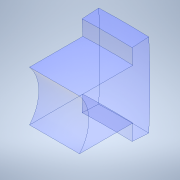
# Autodesk Inventor part: shank_2
Saved by Autodesk Inventor 2020.2 (Build 242310000, 310)
## iProperties
Created: 2021-01-30
Part Number: shank_2
Material: Generic
Document SubType Name: Modeling
Designer: DELL
Density: 1 g/cm^3
Appearance: Clear - Blue
Author: DELL
Autodesk Inventor part; units mm, degrees
ref_plane "XZ Plane" through (0, 0, 0) normal (0, 1, 0) x (-1, 0, 0)
ref_plane "XY Plane" through (0, 0, 0) normal (0, 0, 1) x (1, 0, 0)
ref_plane "UCS1: YZ Plane" through (0, 0, 0) normal (1, 0, 0) x (0, 1, 0)
sketch "Sketch17" plane through (0, 0, 0) normal (1, 0, 0) x (0, 1, 0)
  line L0 (-199.6617, 0) -> (149.874, 0) construction
  line L1 (0, -332.0076) -> (0, 872.0459) projected
  circle A0 centre (0, 0) radius 40
  circle A1 centre (0, 0) radius 46
  arc A2 (-58.5378, -97.8172) -> (58.5378, -97.8172) centre (0, 700.0382) ccw
  arc A3 (-60, -117.7468) -> (60, -117.7468) centre (0, 680) ccw
  line L2 (58.5378, -97.8172) -> (60, -117.7468)
  line L3 (-60, -117.7468) -> (-58.5378, -97.8172)
  line L4 (-30, -34.8712) -> (-30, -99.9618)
  line L5 (-30, -99.9618) -> (30, -99.9618)
  line L6 (30, -99.9618) -> (30, -34.8712)
  line L7 (-48.7654, -98.4741) -> (-50, -118.436)
  line L8 (48.7654, -98.4741) -> (50, -118.436)
  line L9 (-50, -118.436) -> (29.9324, -123.4415) construction
  line L10 (-48.7654, -98.4741) -> (31.1746, -103.3561) construction
  line L11 (-49.3827, -108.455) -> (42.5615, -114.1415) construction
  arc A4 (27.1283, -83.9618) -> (26, -99.9618) centre (99.9403, -97.1362) ccw
  arc A5 (27.1283, -83.9618) -> (30, -51.9618) centre (-149.7281, -51.9618) ccw
  point P0 (0, -120)
  point P1 (0, -99.9618)
  point P2 (0, -120)
  point P3 (0, -46)
  point P4 (0, -99.9618)
  dimension "d173" = 92
  dimension "d174" = 80
  dimension "d224" = 60
  dimension "d229" = 120
  dimension "d230" = 800
  dimension "d231" = 19.9831
  dimension "d232" = 100
  dimension "d233" = 10
  dimension "d235" = 800
  dimension "d241" = 20
  dimension "d242" = 18.7654
  dimension "d243" = 16
  dimension "d244" = 32
  dimension "d245" = 26
  constraints: 20 end point, 16 point on circle, 6 centre point, 5 tangent, 4 point on line, 3 perpendicular, 2 coincident, 1 equal length, 1 line through centre, 1 midpoint, 1 vertical, 5 other
  measures "d173" diameter of A1
  measures "d174" diameter of A0
  measures "d224" distance of L4.end L5.end
  measures "d229" distance from line of point (0, -120) L0
  measures "d230" radius of A3
  measures "d231" distance of L2.start L2.end
  measures "d232" diameter of L7.end L1
  measures "d233" horizontal distance of L3.start L7.end
  measures "d235" radius of A2
  measures "d241" distance of L8.start L8.end
  measures "d242" distance from line of L6 L8.start
  measures "d243" vertical distance of A4.end A4.start
  measures "d244" vertical distance of A4.start A5.end
  measures "d245" distance from line of A4.end L1
sketch "Sketch16" plane through (0, 0, 0) normal (1, 0, 0) x (0, 1, 0)
  circle A0 centre (0, 0) radius 40
  circle A1 centre (0, 0) radius 48.5
  line L0 (0, -201.7) -> (0, 90.2) construction
  line L1 (0, -160) -> (0, -48.5)
  line L2 (30, -38.1084) -> (30, -103.6436)
  line L3 (30, -103.6436) -> (25, -132)
  line L4 (25, -132) -> (50, -132)
  line L5 (50, -132) -> (50, -160)
  line L6 (50, -160) -> (0, -160)
  dimension "d156" = 97
  dimension "d157" = 80
  dimension "d202" = 28
  dimension "d203" = 60
  dimension "d204" = 50
  dimension "d206" = 160
  dimension "d209" = 50
  dimension "d210" = 80
  dimension "d211" = 28.7938
  constraints: 12 end point, 2 centre point, 2 coincident, 2 horizontal, 2 point on circle, 2 point on line, 2 vertical
  measures "d156" diameter of A1
  measures "d157" diameter of A0
  measures "d202" distance of L4.end L5.end
  measures "d203" diameter of L2 L0
  measures "d204" distance of L5.end L1.start
  measures "d206" distance from line of point (0, 0) L6
  measures "d209" diameter of L3.end L0
  measures "d210" angle of L4 L3
  measures "d211" distance of L2.end L3.end
revolve "Revolution2" add sketch "Sketch17" angle 360 about axis through (0, 0, -10) along (0, 0, 1) contours L1 L5 L6 A2 L8 A3 | A2 A4 L5 | L8 A2 L2 A3 | A2 L6 L5 A4
ref_plane "Work Plane7" through (0, -48.7654, -98.4741) normal (0, -0.998093, 0.0617284) x (0, -0.0617284, -0.998093)
split "Split2" plane through (0, -48.7654, -98.4741) removes the side toward (0, -0.998093, 0.0617284)
ref_plane "Work Plane8" through (0, 48.7654, -98.4741) normal (0, -0.998093, -0.0617284) x (0, 0.0617284, -0.998093)
split "Split3" plane through (0, 48.7654, -98.4741) removes the side toward (0, 0.998093, 0.0617284)
ref_plane "Work Plane9" through (-30, 0, 0) normal (1, 0, 0) x (0, 1, 0)
split "Split4" plane through (-30, 0, 0) removes the side toward (-1, 0, 0)
ref_plane "Work Plane10" through (30, 0, 0) normal (1, 0, 0) x (0, 1, 0)
split "Split5" plane through (30, 0, 0) removes the side toward (1, 0, 0)
extrude "Extrusion17" add sketch "Sketch17" along normal mid plane 60 contours L1 A1 L6 A5 A4 A2 | A2 A4 L5 | A4 A5 L6 A2 | A2 L6 L5 A4
fillet "Fillet16" [suppressed]
mirror "Mirror4" about plane through (0, 0, 0) normal (0, 1, 0) of "Extrusion17"
body "Solid1"
body "Solid8"
